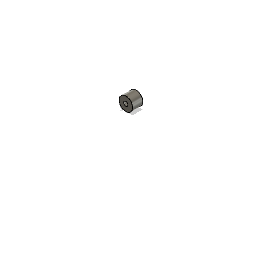
Slip Ring (1) (Autodesk Fusion 360 design; units mm, degrees)
Autodesk Fusion 360 part; units mm, degrees
sketch "Sketch1" plane through (58.1946, -67.3751, 0) normal (0, 0, -1) x (-0.856164, -0.516704, 0)
  circle A0 centre (-50.7749, 52.139) radius 1.5
  circle A1 centre (-20.8092, 70.2236) radius 1.5
  circle A2 centre (-66.6263, 112.0685) radius 1.5
  line L0 (-45.881, 51.3777) -> (-44.1107, 59.8757)
  arc A3 (-43.6798, 60.5082) -> (-44.1107, 59.8757) centre (-43.1318, 59.6718) ccw
  line L1 (-43.6798, 60.5082) -> (-43.6485, 60.5279)
  line L2 (-43.6485, 60.5279) -> (-31.5527, 67.8278)
  arc A4 (-30.7959, 67.9424) -> (-31.5527, 67.8278) centre (-31.036, 66.9716) ccw
  line L3 (-30.7959, 67.9424) -> (-30.7602, 67.9329)
  line L4 (-30.7602, 67.9329) -> (-22.4164, 65.5388)
  arc A5 (-22.4164, 65.5388) -> (-21.656, 65.6253) centre (-22.1406, 66.4999) ccw
  line L5 (-21.656, 65.6253) -> (-21.624, 65.6438)
  line L6 (-21.624, 65.6438) -> (-11.3612, 71.8376)
  arc A6 (-11.3612, 71.8376) -> (-10.8802, 72.6259) centre (-11.8779, 72.6937) ccw
  line L7 (-10.8802, 72.6259) -> (-10.8781, 72.7126)
  arc A7 (-57.6044, 44.5093) -> (-56.681, 44.4906) centre (-57.1248, 45.3869) ccw
  line L8 (-56.681, 44.4906) -> (-56.608, 44.5307)
  line L9 (-56.608, 44.5307) -> (-46.3433, 50.7255)
  arc A8 (-46.3433, 50.7255) -> (-45.8892, 51.3416) centre (-46.86, 51.5817) ccw
  line L10 (-45.8892, 51.3416) -> (-45.881, 51.3777)
  circle A9 centre (42.0163, 114.085) radius 3.429
  circle A10 centre (42.0163, 114.085) radius 10.922
  circle A11 centre (-29.6439, 101.6258) radius 0.175
  circle A12 centre (-32.44, 103.1128) radius 0.175
  line L11 (-10.8781, 72.7126) -> (-19.7385, 128.7003)
  arc A13 (-19.7385, 128.7003) -> (-20.4978, 129.6521) centre (-20.7384, 128.6815) ccw
  line L12 (-20.4978, 129.6521) -> (-20.5833, 129.6693)
  arc A14 (-20.5833, 129.6693) -> (-20.7572, 129.6813) centre (-27.8333, 25.3987) ccw
  line L13 (-20.7572, 129.6813) -> (-20.7899, 129.6801)
  arc A15 (-20.7899, 129.6801) -> (-97.8435, 87.9507) centre (-14.5722, 26.1945) ccw
  line L14 (-97.8435, 87.9507) -> (-102.9093, 80.4579)
  line L15 (-102.9093, 80.4579) -> (-104.2217, 78.2605)
  arc A16 (-104.2217, 78.2605) -> (-103.8712, 76.8901) centre (-103.3613, 77.7505) ccw
  line L16 (-103.8712, 76.8901) -> (-103.8412, 76.8733)
  line L17 (-103.8412, 76.8733) -> (-57.6044, 44.5093)
  circle A17 centre (-41.6146, 118.6098) radius 0.508
  circle A18 centre (-31.0686, 102.0684) radius 0.508
  circle A19 centre (-35.0525, 107.7365) radius 0.508
  circle A20 centre (-29.8174, 99.858) radius 0.508
  circle A21 centre (-38.9897, 114.2605) radius 0.508
  circle A22 centre (-27.3151, 95.4371) radius 0.508
  circle A23 centre (-36.3649, 109.9112) radius 0.508
  circle A24 centre (-28.5662, 97.6476) radius 0.508
  circle A25 centre (-40.3022, 116.4352) radius 0.508
  circle A26 centre (-25.701, 78.5116) radius 0.508
  circle A27 centre (-24.8127, 91.0162) radius 0.508
  circle A28 centre (-50.8357, 67.6243) radius 0.175
  circle A29 centre (-26.9407, 80.7285) radius 0.508
  circle A30 centre (-37.6773, 112.0859) radius 0.508
  circle A31 centre (-26.0639, 93.2266) radius 0.508
  circle A32 centre (-54.8206, 90.9408) radius 21.1582
  circle A33 centre (-79.2839, 74.8665) radius 0.508
  circle A34 centre (-81.4585, 73.5541) radius 0.508
  circle A35 centre (-85.8078, 70.9293) radius 0.508
  circle A36 centre (-83.6332, 72.2417) radius 0.508
  circle A37 centre (-82.7709, 75.7288) radius 0.508
  circle A38 centre (-84.9456, 74.4163) radius 0.508
  circle A39 centre (-80.5963, 77.0412) radius 0.508
  circle A40 centre (-87.9825, 69.6168) radius 0.508
  circle A41 centre (-89.2949, 71.7915) radius 0.508
  circle A42 centre (-87.1203, 73.1039) radius 0.508
  dimension "d785_1" = 6.858
  dimension "d786_1" = 21.844
  constraint concentric A9 A10
  measures "d785_1" diameter of A9
  measures "d786_1" diameter of A10
extrude "Extrude1" add sketch "Sketch1" along normal blind 16.764 contours A10 makes body 1
sketch "Sketch2" plane through (0, 0, -16.764) normal (0, 0, -1) x (-1, 0, 0)
  circle A0 centre (36.7264, 8.5904) radius 3.429
  circle A1 centre (36.7264, 8.5904) radius 10.922
sketch "Sketch3" plane through (-36.7264, 8.5904, -16.764) normal (0, 0, -1) x (-1, 0, 0)
  circle A0 centre (-0.7703, -4.1791) radius 0.3302
  circle A1 centre (-1.4308, -3.9501) radius 0.3302
  circle A2 centre (-2.0913, -3.7211) radius 0.3302
  circle A3 centre (-2.7078, -3.3865) radius 0.3302
  circle A4 centre (-0.0658, -4.2671) radius 0.3302
  circle A5 centre (0.6212, -4.2143) radius 0.3302
  point P0 (-0.7703, -4.1791)
  dimension "d789_1" = 0.6604
  dimension "d790_1" = 0.6604
  dimension "d791_1" = 0.6604
  dimension "d792_1" = 0.6604
  dimension "d793_1" = 0.6604
  dimension "d794_1" = 0.6604
  measures "d789_1" diameter of A0
  measures "d790_1" diameter of A1
  measures "d791_1" diameter of A2
  measures "d792_1" diameter of A3
  measures "d793_1" diameter of A4
  measures "d794_1" diameter of A5
extrude "Extrude2" add sketch "Sketch3" along normal blind 4.4704 bodies 1
sketch "Sketch4" plane through (0, 0, 0) normal (0, 0, 1) x (1, 0, 0)
  circle A0 centre (-36.7264, 8.5904) radius 3.429
  circle A1 centre (-36.7264, 8.5904) radius 10.922
  circle A2 centre (-42.7214, 103.9048) radius 0.3302
  circle A3 centre (-41.9869, 103.8721) radius 0.3302
  circle A4 centre (-41.1872, 103.9048) radius 0.3302
  circle A5 centre (-41.1872, 124.2406) radius 0.3302
  circle A6 centre (-41.9869, 124.208) radius 0.3302
  circle A7 centre (-42.7214, 124.2406) radius 0.3302
  dimension "d797_1" = 0.6604
  dimension "d798_1" = 0.6604
  dimension "d799_1" = 0.6604
  dimension "d800_1" = 0.6604
  dimension "d801_1" = 0.6604
  dimension "d802_1" = 0.6604
  measures "d797_1" diameter of A2
  measures "d798_1" diameter of A3
  measures "d799_1" diameter of A4
  measures "d800_1" diameter of A7
  measures "d801_1" diameter of A6
  measures "d802_1" diameter of A5
extrude "Extrude3" add sketch "Sketch4" along normal blind 3.175 contours A2 | A3 | A4 | A5 | A6 | A7 bodies 1 makes body 2 at (-42.4014, 124.3221, 2.1167) makes body 3 at (-42.4014, 103.9862, 2.1167) makes body 4 at (-41.6669, 124.2894, 2.1167) makes body 5 at (-40.8672, 103.9863, 2.1167) makes body 6 at (-41.6669, 103.9536, 2.1167) makes body 7 at (-40.8672, 124.3221, 2.1167)
sketch "sketch 1354" plane through (53.5411, -109.8708, 62.738) normal (0, -1, 0) x (-0.030286, 0, 0.999541)
  circle A0 centre (54.2175, 93.9584) radius 10.922
extrude "Extrude4" cut sketch "sketch 1354" against normal up to surface (213.7582 mm away) bodies 7 1 5 4 6 2 3
